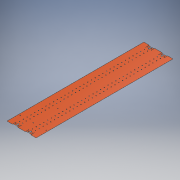
# Autodesk Inventor part: Skin NPS 18
Saved by Autodesk Inventor 2019 (Build 230136000, 136)
## iProperties
Created: 2016-08-10
Part Number: Skin NPS 18
Material: Rubber, Silicone
Document SubType Name: Modeling
Designer: IEUser
Density: 1.25 g/cm^3
Appearance: Rubber - Black
Author: IEUser
Autodesk Inventor part; units mm, degrees
ref_plane "YZ Plane" through (0, 0, 0) normal (1, 0, 0) x (0, 1, 0)
ref_plane "XZ Plane" through (0, 0, 0) normal (0, 1, 0) x (-1, 0, 0)
ref_plane "XY Plane" through (0, 0, 0) normal (0, 0, 1) x (1, 0, 0)
sketch "Skin Scheme" plane through (0, 0, 0) normal (0, 1, 0) x (-1, 0, 0)
  line L0 (1134.5, -212) -> (-1134.5, -212)
  line L1 (-1134.5, -212) -> (-1134.5, 212)
  line L2 (-1134.5, 212) -> (1134.5, 212)
  line L3 (1134.5, 212) -> (1134.5, -212)
  circle A0 centre (962.5, -116) radius 5
  circle A1 centre (962.5, -72) radius 5
  circle A2 centre (962.5, 72) radius 5
  circle A3 centre (962.5, 116) radius 5
  circle A4 centre (907.5, -116) radius 5
  circle A5 centre (907.5, -72) radius 5
  circle A6 centre (907.5, 72) radius 5
  circle A7 centre (907.5, 116) radius 5
  circle A8 centre (852.5, -116) radius 5
  circle A9 centre (852.5, -72) radius 5
  circle A10 centre (852.5, 72) radius 5
  circle A11 centre (852.5, 116) radius 5
  circle A12 centre (797.5, -116) radius 5
  circle A13 centre (797.5, -72) radius 5
  circle A14 centre (797.5, 72) radius 5
  circle A15 centre (797.5, 116) radius 5
  circle A16 centre (742.5, -116) radius 5
  circle A17 centre (742.5, -72) radius 5
  circle A18 centre (742.5, 72) radius 5
  circle A19 centre (742.5, 116) radius 5
  circle A20 centre (687.5, -116) radius 5
  circle A21 centre (687.5, -72) radius 5
  circle A22 centre (687.5, 72) radius 5
  circle A23 centre (687.5, 116) radius 5
  circle A24 centre (632.5, -116) radius 5
  circle A25 centre (632.5, -72) radius 5
  circle A26 centre (632.5, 72) radius 5
  circle A27 centre (632.5, 116) radius 5
  circle A28 centre (577.5, -116) radius 5
  circle A29 centre (577.5, -72) radius 5
  circle A30 centre (577.5, 72) radius 5
  circle A31 centre (577.5, 116) radius 5
  circle A32 centre (522.5, -116) radius 5
  circle A33 centre (522.5, -72) radius 5
  circle A34 centre (522.5, 72) radius 5
  circle A35 centre (522.5, 116) radius 5
  circle A36 centre (467.5, -116) radius 5
  circle A37 centre (467.5, -72) radius 5
  circle A38 centre (467.5, 72) radius 5
  circle A39 centre (467.5, 116) radius 5
  circle A40 centre (412.5, -116) radius 5
  circle A41 centre (412.5, -72) radius 5
  circle A42 centre (412.5, 72) radius 5
  circle A43 centre (412.5, 116) radius 5
  circle A44 centre (357.5, -116) radius 5
  circle A45 centre (357.5, -72) radius 5
  circle A46 centre (357.5, 72) radius 5
  circle A47 centre (357.5, 116) radius 5
  circle A48 centre (302.5, -116) radius 5
  circle A49 centre (302.5, -72) radius 5
  circle A50 centre (302.5, 72) radius 5
  circle A51 centre (302.5, 116) radius 5
  circle A52 centre (247.5, -116) radius 5
  circle A53 centre (247.5, -72) radius 5
  circle A54 centre (247.5, 72) radius 5
  circle A55 centre (247.5, 116) radius 5
  circle A56 centre (192.5, -116) radius 5
  circle A57 centre (192.5, -72) radius 5
  circle A58 centre (192.5, 72) radius 5
  circle A59 centre (192.5, 116) radius 5
  circle A60 centre (137.5, -116) radius 5
  circle A61 centre (137.5, -72) radius 5
  circle A62 centre (137.5, 72) radius 5
  circle A63 centre (137.5, 116) radius 5
  circle A64 centre (82.5, -116) radius 5
  circle A65 centre (82.5, -72) radius 5
  circle A66 centre (82.5, 72) radius 5
  circle A67 centre (82.5, 116) radius 5
  circle A68 centre (27.5, -116) radius 5
  circle A69 centre (27.5, -72) radius 5
  circle A70 centre (27.5, 72) radius 5
  circle A71 centre (27.5, 116) radius 5
  circle A72 centre (-27.5, -116) radius 5
  circle A73 centre (-27.5, -72) radius 5
  circle A74 centre (-27.5, 72) radius 5
  circle A75 centre (-27.5, 116) radius 5
  circle A76 centre (-82.5, -116) radius 5
  circle A77 centre (-82.5, -72) radius 5
  circle A78 centre (-82.5, 72) radius 5
  circle A79 centre (-82.5, 116) radius 5
  circle A80 centre (825, 0) radius 5
  circle A81 centre (825, -188) radius 5
  circle A82 centre (825, 188) radius 5
  circle A83 centre (467.5, 0) radius 5
  circle A84 centre (-137.5, -116) radius 5
  circle A85 centre (-137.5, -72) radius 5
  circle A86 centre (-137.5, 72) radius 5
  circle A87 centre (-137.5, 116) radius 5
  circle A88 centre (-192.5, -116) radius 5
  circle A89 centre (-192.5, -72) radius 5
  circle A90 centre (-192.5, 72) radius 5
  circle A91 centre (-192.5, 116) radius 5
  circle A92 centre (-247.5, -116) radius 5
  circle A93 centre (-247.5, -72) radius 5
  circle A94 centre (-247.5, 72) radius 5
  circle A95 centre (-247.5, 116) radius 5
  circle A96 centre (-302.5, -116) radius 5
  circle A97 centre (-302.5, -72) radius 5
  circle A98 centre (-302.5, 72) radius 5
  circle A99 centre (-302.5, 116) radius 5
  circle A100 centre (-357.5, -116) radius 5
  circle A101 centre (-357.5, -72) radius 5
  circle A102 centre (-357.5, 72) radius 5
  circle A103 centre (-357.5, 116) radius 5
  circle A104 centre (-412.5, -116) radius 5
  circle A105 centre (-412.5, -72) radius 5
  circle A106 centre (-412.5, 72) radius 5
  circle A107 centre (-412.5, 116) radius 5
  circle A108 centre (-467.5, -116) radius 5
  circle A109 centre (-467.5, -72) radius 5
  circle A110 centre (-467.5, 72) radius 5
  circle A111 centre (-467.5, 116) radius 5
  circle A112 centre (-522.5, -116) radius 5
  circle A113 centre (-522.5, -72) radius 5
  circle A114 centre (-522.5, 72) radius 5
  circle A115 centre (-522.5, 116) radius 5
  circle A116 centre (-577.5, -116) radius 5
  circle A117 centre (-577.5, -72) radius 5
  circle A118 centre (-577.5, 72) radius 5
  circle A119 centre (-577.5, 116) radius 5
  circle A120 centre (-632.5, -116) radius 5
  circle A121 centre (-632.5, -72) radius 5
  circle A122 centre (-632.5, 72) radius 5
  circle A123 centre (-632.5, 116) radius 5
  circle A124 centre (-687.5, -116) radius 5
  circle A125 centre (-687.5, -72) radius 5
  circle A126 centre (-687.5, 72) radius 5
  circle A127 centre (-687.5, 116) radius 5
  circle A128 centre (-742.5, -116) radius 5
  circle A129 centre (-742.5, -72) radius 5
  circle A130 centre (-742.5, 72) radius 5
  circle A131 centre (-742.5, 116) radius 5
  circle A132 centre (-797.5, -116) radius 5
  circle A133 centre (-797.5, -72) radius 5
  circle A134 centre (-797.5, 72) radius 5
  circle A135 centre (-797.5, 116) radius 5
  circle A136 centre (-852.5, -116) radius 5
  circle A137 centre (-852.5, -72) radius 5
  circle A138 centre (-852.5, 72) radius 5
  circle A139 centre (-852.5, 116) radius 5
  circle A140 centre (-907.5, -116) radius 5
  circle A141 centre (-907.5, -72) radius 5
  circle A142 centre (-907.5, 72) radius 5
  circle A143 centre (-907.5, 116) radius 5
  circle A144 centre (-962.5, -116) radius 5
  circle A145 centre (-962.5, -72) radius 5
  circle A146 centre (-962.5, 72) radius 5
  circle A147 centre (-962.5, 116) radius 5
  point P0 (0, 0)
  dimension "d0" = 2269
  dimension "d1" = 1134.5
  dimension "d2" = 424
  dimension "d3" = 212
  dimension "d4" = 10
  dimension "d5" = 172
  dimension "d6" = 96
  dimension "d9" = 44
  dimension "d16" = 188
  dimension "d19" = 55
  dimension "d61" = 27.5
  dimension "d62" = 72
  dimension "d63" = 72
  dimension "d64" = 27.5
  dimension "d65" = 72
  dimension "d66" = 27.5
  dimension "d67" = 10
  dimension "d68" = 10
  dimension "d69" = 10
  dimension "d70" = 495
  dimension "d71" = 0
  dimension "d72" = 10
  constraints: 148 centre point, 8 end point, 2 horizontal, 2 parallel, 2 vertical, 1 perpendicular, 286 other
  measures "d0" distance of L0.start L0.end
  measures "d1" distance from line of point (0, 0) L3
  measures "d2" distance of L2.end L0.start
  measures "d3" distance from line of point (0, 0) L0
  measures "d4" diameter of A0
  measures "d5" distance from line of L3 A0.centre
  measures "d6" distance from line of L0 A0.centre
  measures "d9" distance of A0.centre A1.centre
  measures "d16" distance of A0.centre A2.centre
  measures "d19" distance of A0.centre A4.centre
  measures "d61" horizontal distance of A9.centre A80.centre
  measures "d62" vertical distance of A9.centre A80.centre
  measures "d63" vertical distance of A8.centre A81.centre
  measures "d64" horizontal distance of A81.centre A8.centre
  measures "d65" vertical distance of A11.centre A82.centre
  measures "d66" horizontal distance of A11.centre A82.centre
  measures "d67" diameter of A82
  measures "d68" diameter of A80
  measures "d69" diameter of A81
  measures "d70" horizontal distance of A83.centre A1.centre
  measures "d71" vertical distance of point (0, 0) A83.centre
  measures "d72" diameter of A83
extrude "Skin Body" add sketch "Skin Scheme" along normal blind 1
sketch "Feature Cut Outline" plane through (0, 1, 0) normal (0, 1, 0) x (1, 0, 0)
  circle A0 centre (-962.5, 116) radius 5 projected
  circle A1 centre (-962.5, 72) radius 5 projected
  line L0 (-1144.5, 134) -> (-984.5, 134)
  line L1 (-984.5, 134) -> (-984.5, 99)
  line L2 (-984.5, 99) -> (-944.5, 99)
  line L3 (-944.5, 99) -> (-939.5, 94)
  line L4 (-939.5, 94) -> (-944.5, 84)
  line L5 (-944.5, 84) -> (-984.5, 84)
  line L6 (-984.5, 84) -> (-984.5, 54)
  line L7 (-984.5, 54) -> (-1144.5, 54)
  line L8 (-1144.5, 54) -> (-1144.5, 134)
  line L9 (-1134.5, 212) -> (-1134.5, -212) projected
  point P0 (0, 0)
  dimension "d33" = 18
  dimension "d34" = 22
  dimension "d35" = 18
  dimension "d36" = 5
  dimension "d37" = 10
  dimension "d38" = 5
  dimension "d39" = 5
  dimension "d40" = 10
  dimension "d41" = 45
  dimension "d42" = 22
  constraints: 18 end point, 3 perpendicular, 2 parallel, 1 collinear, 1 horizontal
  measures "d33" distance from line of A0.centre L0
  measures "d34" distance from line of L1 A0.centre
  measures "d35" distance from line of A1.centre L7
  measures "d36" distance from line of L3.end L2
  measures "d37" distance from line of L3.end L5
  measures "d38" horizontal distance of L4.end L3.end
  measures "d39" horizontal distance of L2.end L3.end
  measures "d40" distance between parallel lines of L9 L8
  measures "d41" distance from line of L6 L3.end
  measures "d42" vertical distance of A1.centre L3.end
extrude "Feature Cut" cut sketch "Feature Cut Outline" along normal through all both and the other way through all contours L0 L9 L7 L8 | L0 L1 L2 L3 L4 L5 L6 L7 L9
mirror "Feature Cut Side Mirror" about plane through (0, 0, 0) normal (0, 0, 1) of "Feature Cut"
mirror "Feature Cut Mirror" about plane through (0, 0, 0) normal (1, 0, 0) of "Feature Cut", "Feature Cut Side Mirror"
sketch "End Cut Outline" plane through (0, 1, 0) normal (0, 1, 0) x (1, 0, 0)
  line L0 (-994.5, 222) -> (-1144.5, 222)
  line L1 (-1144.5, 222) -> (-1144.5, -222)
  line L2 (-1144.5, -222) -> (-994.5, -222)
  line L3 (-994.5, -222) -> (-994.5, 222)
  line L4 (-1134.5, 212) -> (-1134.5, 134) projected
  line L5 (1134.5, 212) -> (-1134.5, 212) projected
  line L6 (-1134.5, -212) -> (1134.5, -212) projected
  point P0 (0, 0)
  dimension "d45" = 10
  dimension "d46" = 10
  dimension "d47" = 10
  dimension "d48" = 140
  constraints: 8 end point, 2 parallel, 1 horizontal, 1 perpendicular
  measures "d45" distance between parallel lines of L4 L1
  measures "d46" distance between parallel lines of L5 L0
  measures "d47" distance between parallel lines of L2 L6
  measures "d48" distance between parallel lines of L4 L3
extrude "End Cut" cut sketch "End Cut Outline" along normal through all both and the other way through all
mirror "End Cut Mirror" about plane through (0, 0, 0) normal (1, 0, 0) of "End Cut"
sketch "Slot Cut Outline" plane through (0, 1, 0) normal (0, 1, 0) x (1, 0, 0)
  line L0 (-942.5, 55) -> (-994.5, 55)
  line L1 (-994.5, 55) -> (-994.5, 54)
  line L2 (-994.5, 54) -> (-942.5, 54)
  line L3 (-942.5, 54) -> (-942.5, 55)
  line L4 (-984.5, 54) -> (-994.5, 54) projected
  line L5 (-994.5, 54) -> (-994.5, -54) projected
  line L6 (-984.5, 84) -> (-984.5, 54) projected
  line L7 (-994.5, 134) -> (-942.5, 134)
  line L8 (-942.5, 134) -> (-942.5, 133)
  line L9 (-942.5, 133) -> (-994.5, 133)
  line L10 (-994.5, 133) -> (-994.5, 134)
  line L11 (-994.5, 134) -> (-984.5, 134) projected
  line L12 (-984.5, 134) -> (-984.5, 99) projected
  line L13 (-994.5, 212) -> (-994.5, 134) projected
  point P0 (0, 0)
  dimension "d51" = 0
  dimension "d52" = 1
  dimension "d53" = 0
  dimension "d54" = 42
  dimension "d55" = 0
  dimension "d56" = 1
  dimension "d57" = 42
  dimension "d58" = 0
  constraints: 16 end point, 4 parallel, 2 horizontal, 2 perpendicular
  measures "d51" distance between parallel lines of L4 L2
  measures "d52" distance of L2.end L0.start
  measures "d53" distance between parallel lines of L5 L1
  measures "d54" distance between parallel lines of L6 L3
  measures "d55" distance between parallel lines of L11 L7
  measures "d56" distance of L7.end L8.end
  measures "d57" distance between parallel lines of L12 L8
  measures "d58" distance between parallel lines of L13 L10
extrude "Slot Cut" cut sketch "Slot Cut Outline" along normal through all both and the other way through all
mirror "Slot Cut Side Mirror" about plane through (0, 0, 0) normal (0, 0, 1) of "Slot Cut"
mirror "Slot Cut Mirror" about plane through (0, 0, 0) normal (1, 0, 0) of "Slot Cut", "Slot Cut Side Mirror"
equation "\"d1\" = 0.5 * d0"
equation "\"d3\" = 0.5 * d2"
equation "\"d61\" = 0.5 * d19"
equation "\"d62\" = -0.5 * d9 + 0.5 * d16"
equation "\"d63\" = d62"
equation "\"d64\" = d61"
equation "\"d65\" = d62"
equation "\"d66\" = d61"
equation "\"d67\" = d4"
equation "\"d68\" = d4"
equation "\"d69\" = d4"
equation "\"d56\" = d52"
equation "\"d57\" = d54"
body "Solid1"
